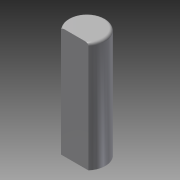
# Autodesk Inventor part: axe
Saved by Autodesk Inventor 2014 SP2 (Build 180246200, 246)
## iProperties
Created: 2015-03-17
Part Number: axe
Material: Acier
Document SubType Name: Modeling
Designer: sd
Density: 7.85 g/cm^3
Appearance: Acier
Mass: 0.444224 g
Surface Area: 0.942013 cm^2
Volume: 0.056589 cm^3
Author: sd
Autodesk Inventor part; units mm, degrees
ref_plane "YZ Plane" through (0, 0, 0) normal (1, 0, 0) x (0, 1, 0)
ref_plane "XZ Plane" through (0, 0, 0) normal (0, 1, 0) x (-1, 0, 0)
ref_plane "XY Plane" through (0, 0, 0) normal (0, 0, 1) x (1, 0, 0)
sketch "Esquisse2" plane through (0, 0, 0) normal (0, 0, 1) x (1, 0, 0)
  circle A0 centre (0, 0) radius 1.5
  line L0 (-1.118, -1) -> (1.118, -1)
  dimension "d2" = 3
  dimension "d3" = 0.5
  constraints: 2 end point, 2 point on circle, 1 centre point, 1 coincident, 1 horizontal
  measures "d2" diameter of A0
  measures "d3" distance edge to line of A0 L0
extrude "Extrusion1" add sketch "Esquisse2" along normal blind 9 contours A0 L0 picked at (0.0594, -0.1702)
fillet "Congé1" radius 0.2 1 edges at (0, 1.5, 9)
